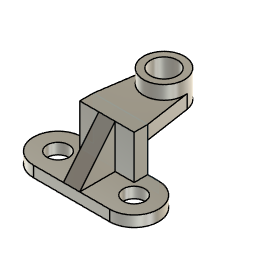
EDM 2.2 (Autodesk Fusion 360 design; units mm, degrees)
part number: 2025-09-15-08-01-47-290
Autodesk Fusion 360 part; units mm, degrees
sketch "Sketch1" plane through (0, 0, 0) normal (0, 0, 1) x (1, 0, 0)
  line L0 (28, -18) -> (-28, -18)
  line L1 (-28, 18) -> (28, 18)
  line L2 (28, -18) -> (-28, 18) construction
  line L3 (-28, -18) -> (28, 18) construction
  circle A0 centre (-28, 0) radius 8
  circle A1 centre (28, 0) radius 8
  arc A2 (-28, 18) -> (-28, -18) centre (-28, 0) ccw
  arc A3 (28, -18) -> (28, 18) centre (28, 0) ccw
  dimension "d1" = 56
  dimension "d2" = 36
  dimension "d3" = 36
  dimension "d4" = 36
  dimension "d5" = 16
  dimension "d6" = 16
  constraint horizontal L0
  constraint parallel L0 L1
  constraint coincident L2 origin
  constraint coincident L3 origin
  constraint concentric A0 A2
  constraint concentric A1 A3
  measures "d1" distance of L1.start L1.end
  measures "d2" distance of L0.end L1.start
  measures "d3" diameter of A2
  measures "d4" diameter of A3
  measures "d5" diameter of A0
  measures "d6" diameter of A1
extrude "Extrude1" add sketch "Sketch1" along normal blind 8
sketch "Sketch2" plane through (0, 0, 8) normal (0, 0, 1) x (-1, 0, 0)
  circle A0 centre (-28, 0) radius 8
  circle A1 centre (28, 0) radius 8
  arc A2 (28, -18) -> (28, 18) centre (28, 0) ccw
  line L0 (28, 18) -> (-28, 18)
  arc A3 (-28, 18) -> (-28, -18) centre (-28, 0) ccw
  line L1 (-28, -18) -> (28, -18)
  line L2 (-20, -18) -> (-20, -8)
  line L3 (-20, -8) -> (20, -8)
  line L4 (20, -8) -> (20, -18)
  dimension "d9" = 40
  constraint parallel L2 L4
  constraint coincident L1 L2.start
  constraint coincident L1 L4.end
extrude "Extrude2" add sketch "Sketch2" along normal blind 32 contours L1 L2 L3 L4
sketch "Sketch3" plane through (0, 18, 0) normal (0, 1, 0) x (-1, 0, 0)
  line L0 (-28, 0) -> (28, 0)
  line L1 (28, 0) -> (28, 8)
  line L2 (28, 8) -> (20, 8)
  line L3 (20, 8) -> (20, 40)
  line L4 (20, 40) -> (-20, 40)
  line L5 (-20, 40) -> (-20, 8)
  line L6 (-20, 8) -> (-28, 8)
  line L7 (-28, 8) -> (-28, 0)
sketch "Sketch4" plane through (0, 0, 40) normal (0, 0, 1) x (-1, 0, 0)
  line L0 (-20, -18) -> (20, -18)
  line L1 (20, -18) -> (20, -8)
  line L2 (20, -8) -> (-20, -8)
  line L3 (-20, -8) -> (-20, -18)
  circle A0 centre (0, -50) radius 15
  circle A1 centre (0, -50) radius 10
  line L4 (20, -18) -> (14.832, -52.2387)
  line L5 (-20, -18) -> (-14.832, -52.2387)
  dimension "d13" = 30
  dimension "d14" = 20
  dimension "d15" = 32
  constraint concentric A0 A1
  constraint coincident L0.end L1.start
  constraint coincident L0.start L3.end
  constraint tangent A0 L4
  constraint tangent A0 L5
  constraint coincident A0 L4.end
  constraint coincident A0 L5.end
  measures "d13" diameter of A0
  measures "d14" diameter of A1
  measures "d15" vertical distance of L0.start A0.centre
extrude "Extrude3" add sketch "Sketch4" against normal blind 10 contours L0 A0 L4 L5 | A0
sketch "Sketch5" plane through (0, 0, 40) normal (0, 0, 1) x (-1, 0, 0)
  circle A0 centre (0, -50) radius 10
  line L0 (20, -18) -> (20, -8)
  line L1 (20, -8) -> (-20, -8)
  line L2 (-20, -8) -> (-20, -18)
  line L3 (-20, -18) -> (-14.832, -52.2387)
  arc A1 (-14.832, -52.2387) -> (14.832, -52.2387) centre (0, -50) ccw
  line L4 (14.832, -52.2387) -> (20, -18)
  circle A2 centre (0, -50) radius 15
  dimension "d18" = 30
  constraint concentric A0 A2
  measures "d18" diameter of A2
extrude "Extrude4" add sketch "Sketch5" along normal blind 10 contours A1 A2
ref_plane "WorkPlane1" through (0, 13, 24) normal (-1, 0, 0) x (0, -1, 0)
sketch "Sketch6" plane through (0, 0, 0) normal (-1, 0, 0) x (0, -1, 0)
  line L0 (18, 8) -> (-8, 8)
  line L1 (-8, 8) -> (-8, 40)
  line L2 (-8, 40) -> (18, 8)
  point P0 (-8, 40)
  point P1 (-8, 8)
  point P2 (18, 8)
  constraint coincident P2 L0.start
  constraint coincident P1 L0.end
  constraint coincident P0 L1.end
extrude "Extrude5" add sketch "Sketch6" along normal blind 6 and the other way blind 6
